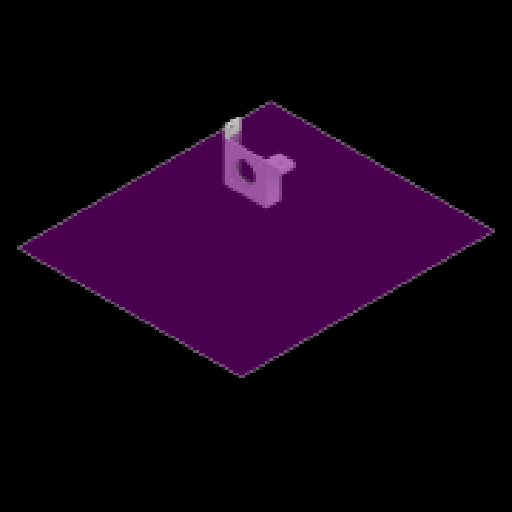
# Autodesk Inventor part: PancakeNema17MotorMount
Saved by Autodesk Inventor 2025 (Build 290162000, 162)
## iProperties
Created: 2024-11-19
Part Number: PancakeNema17MotorMount
Material: Generic
Document SubType Name: Modeling
Designer: Trevor
Density: 1 g/cm^3
Appearance: Default
Author: Trevor
Autodesk Inventor part; units mm, degrees
ref_plane "YZ Plane" through (0, 0, 0) normal (1, 0, 0) x (0, 1, 0)
ref_plane "XZ Plane" through (0, 0, 0) normal (0, 1, 0) x (-1, 0, 0)
ref_plane "XY Plane" through (0, 0, 0) normal (0, 0, 1) x (1, 0, 0)
sketch "Sketch1" plane through (0, 0, 0) normal (0, 0, 1) x (1, 0, 0)
  line L0 (-20, 16.5858) -> (-16.5858, 20) projected
  line L1 (-20, -16.5858) -> (-20, 16.5858) projected
  line L2 (-16.5858, -20) -> (-20, -16.5858) projected
  line L3 (16.5858, -20) -> (-16.5858, -20) projected
  line L4 (20, -16.5858) -> (16.5858, -20) projected
  line L5 (20, 16.5858) -> (20, -16.5858) projected
  line L6 (16.5858, 20) -> (20, 16.5858) projected
  line L7 (-16.5858, 20) -> (16.5858, 20) projected
  circle A0 centre (15.5, -15.5) radius 1.5 projected
  circle A1 centre (-15.5, 15.5) radius 1.5 projected
  circle A2 centre (-15.5, -15.5) radius 1.5 projected
  circle A3 centre (15.5, 15.5) radius 1.5 projected
  circle A4 centre (0, 0) radius 11 projected
  circle A5 centre (0, 0) radius 4.9 projected
  line L8 (13.1931, -21.15) -> (-13.1931, -21.15) projected
  line L9 (-21.15, -13.1931) -> (-21.15, 13.1931) projected
  line L10 (21.15, 21.15) -> (-21.15, 21.15)
  line L11 (-21.15, 21.15) -> (-21.15, -21.15)
  line L12 (-21.15, -21.15) -> (21.15, -21.15)
  line L13 (21.15, -21.15) -> (21.15, 21.15)
  line L14 (21.15, 21.15) -> (-21.15, -21.15) construction
  line L15 (-21.15, 21.15) -> (21.15, -21.15) construction
  line L16 (23.15, -23.15) -> (-23.15, -23.15)
  line L17 (-23.15, -23.15) -> (-23.15, 21.15)
  line L18 (23.15, 21.15) -> (23.15, -23.15)
  line L19 (23.15, 21.15) -> (-23.15, 21.15)
  line L20 (-23.15, 21.15) -> (-23.1187, 21.15)
  line L21 (23.15, 21.15) -> (21.15, 21.15)
  line L22 (-13.1931, -21.15) -> (13.1931, -21.15)
  dimension "d0" = 2
  constraints: 26 end point, 3 parallel, 3 point on line, 2 collinear, 2 horizontal, 2 midpoint, 1 perpendicular
  measures "d0" distance between parallel lines of L12 L16
extrude "Extrusion1" add sketch "Sketch1" along normal blind 2 contours L0 L7 L6 L5 L4 L3 L2 L1 | L12 L13 L19 L18 L16 L17 L11 L9 L8 | L8 L12 L11 L9 L10 L13
sketch "Sketch2" plane through (0, 0, 0) normal (0, 0, -1) x (-1, 0, 0)
  line L0 (21, -10) -> (21, 10) projected
  line L1 (-21, 10) -> (-21, -10) projected
  line L2 (-198.65, 21.15) -> (16.15, 21.15) projected
  line L3 (21, -21.15) -> (-21, -21.15)
  line L4 (-21, -21.15) -> (-21, 21.15)
  line L5 (-21, 21.15) -> (21, 21.15)
  line L6 (21, 21.15) -> (21, -21.15)
  line L7 (21, -21.15) -> (-21, 21.15) construction
  line L8 (-21, -21.15) -> (21, 21.15) construction
  line L9 (23.15, -23.15) -> (-23.15, -23.15) projected
  line L10 (-23.15, -23.15) -> (-23.15, 21.15) projected
  line L11 (23.15, 21.15) -> (23.15, -23.15) projected
  line L12 (-23.15, 21.15) -> (23.15, 21.15) projected
  line L13 (21, 21.15) -> (23.15, 21.15)
  line L14 (23.15, 21.15) -> (-21, 21.15)
  line L15 (-21, 21.15) -> (-23.15, 21.15)
  point P0 (0, 0)
  constraints: 18 end point, 3 collinear, 2 midpoint, 2 parallel, 1 horizontal, 1 perpendicular, 1 point on line
ref_plane "Work Plane1" through (-21, -21, -14) normal (0, 0, 1) x (1, 0, 0)
extrude "Extrusion2" add sketch "Sketch2" along normal up to surface (14 mm away) contours L0 L6 L12 L11 L9 L10 L2 L4 L1 L3
sketch "Sketch3" plane through (-23.15, 21.15, 2) normal (0, 1, 0) x (1, 0, 0)
  line L0 (44.15, 2) -> (2.15, 2) projected
  line L1 (2.15, 2) -> (2.15, 16) projected
  line L2 (0, 16) -> (2.15, 16) projected
  line L3 (0, 16) -> (0, 0) projected
  line L4 (46.3, 0) -> (0, 0) projected
  line L5 (46.3, 0) -> (46.3, 16) projected
  line L6 (44.15, 16) -> (46.3, 16) projected
  line L7 (44.15, 2) -> (44.15, 16) projected
  arc A0 (2, -201.375) -> (7, -206.375) centre (7, -201.375) ccw projected
  line L8 (7, -206.375) -> (221.8, -206.375) projected
  arc A1 (221.8, -206.375) -> (226.8, -201.375) centre (221.8, -201.375) ccw projected
  line L9 (226.8, -201.375) -> (226.8, -174.375) projected
  arc A2 (226.8, -174.375) -> (221.8, -169.375) centre (221.8, -174.375) ccw projected
  line L10 (221.8, -169.375) -> (151.8, -169.375) projected
  arc A3 (146.8, -164.375) -> (151.8, -169.375) centre (151.8, -164.375) ccw projected
  line L11 (146.8, -164.375) -> (146.8, 5.625) projected
  arc A4 (151.8, 10.625) -> (146.8, 5.625) centre (151.8, 5.625) ccw projected
  line L12 (151.8, 10.625) -> (221.8, 10.625) projected
  arc A5 (221.8, 10.625) -> (226.8, 15.625) centre (221.8, 15.625) ccw projected
  line L13 (226.8, 15.625) -> (226.8, 42.625) projected
  arc A6 (226.8, 42.625) -> (221.8, 47.625) centre (221.8, 42.625) ccw projected
  line L14 (221.8, 47.625) -> (7, 47.625) projected
  arc A7 (7, 47.625) -> (2, 42.625) centre (7, 42.625) ccw projected
  line L15 (2, 42.625) -> (2, 5) projected
  arc A8 (2, 5) -> (7, 0) centre (7, 5) ccw projected
  line L16 (7, 0) -> (78.6, 0) projected
  arc A9 (83.6, -5) -> (78.6, 0) centre (78.6, -5) ccw projected
  line L17 (83.6, -5) -> (83.6, -153.75) projected
  arc A10 (78.6, -158.75) -> (83.6, -153.75) centre (78.6, -153.75) ccw projected
  line L18 (78.6, -158.75) -> (7, -158.75) projected
  arc A11 (7, -158.75) -> (2, -163.75) centre (7, -163.75) ccw projected
  line L19 (2, -163.75) -> (2, -201.375) projected
  line L20 (2, 5) -> (0, 5)
  circle A12 centre (208.3, 29.125) radius 5 projected
  circle A13 centre (208.3, -187.875) radius 5 projected
  circle A14 centre (20.5, 29.125) radius 5 projected
  circle A15 centre (20.5, -187.875) radius 5 projected
  point P0 (23.15, 2)
  point P1 (2, 16)
  constraints: 2 end point, 1 perpendicular, 1 point on line
ref_plane "Work Plane2" through (-21.15, 33.85, -45.625) normal (0, 1, 0) x (0, 0, 1)
extrude "Extrusion3" add sketch "Sketch3" along normal up to surface (12.7 mm away) contours A8 L4 L3 L20 L1 L0 | L0 L1 A8 | L20 L3 L2 L15
sketch "Sketch4" plane through (-23.15, -23.15, -14) normal (-1, 0, 0) x (0, 0, 1)
  line L0 (0, 0) -> (0, 57) projected
  line L1 (16, 0) -> (16, 57) projected
  line L2 (0, 57) -> (16, 57)
  line L3 (16, 57) -> (16, 44.5)
  line L4 (16, 44.5) -> (0, 44.5)
  line L5 (0, 44.5) -> (0, 57)
  circle A0 centre (8, 50.75) radius 2.5
  point P0 (14, 23.15)
  dimension "d7" = 12.5
  dimension "d8" = 5
  constraints: 8 end point, 2 parallel, 1 centre point, 1 horizontal, 1 perpendicular, 1 point on line
  measures "d7" distance of L2.end L3.end
  measures "d8" diameter of A0
extrude "Extrusion4" cut sketch "Sketch4" against normal blind 2 contours A0
ref_plane "Work Plane3" through (81.25, 21.15, 81.375) normal (0, -1, 0) x (0, 0, 1)
sketch "Sketch5" plane through (81.25, 21.15, 81.375) normal (0, -1, 0) x (0, 0, 1)
  line L0 (-95.375, 58.1) -> (-79.375, 58.1) projected
  line L1 (-95.375, 58.1) -> (-79.375, 58.1) projected
  line L2 (-79.375, 104.4) -> (-79.375, 58.1) projected
  line L3 (-95.375, 104.4) -> (-79.375, 104.4) projected
  line L4 (-95.375, 58.1) -> (-95.375, 104.4) projected
  line L5 (-95.375, 58.1) -> (-79.375, 58.1)
  line L6 (-79.375, 58.1) -> (-79.375, 42.1)
  line L7 (-79.375, 42.1) -> (-95.375, 42.1)
  line L8 (-95.375, 42.1) -> (-95.375, 58.1)
  circle A0 centre (-87.375, 50.1) radius 2.5
  point P0 (-81.375, 81.25)
  dimension "d11" = 16
  dimension "d12" = 16
  dimension "d13" = 5
  constraints: 8 end point, 2 parallel, 1 centre point, 1 horizontal, 1 perpendicular
  measures "d11" distance of L6.end L7.end
  measures "d12" distance of L5.end L6.end
  measures "d13" diameter of A0
extrude "Extrusion6" add sketch "Sketch5" along normal blind 5 contours L0 L6 L7 L8
body "Solid1"
